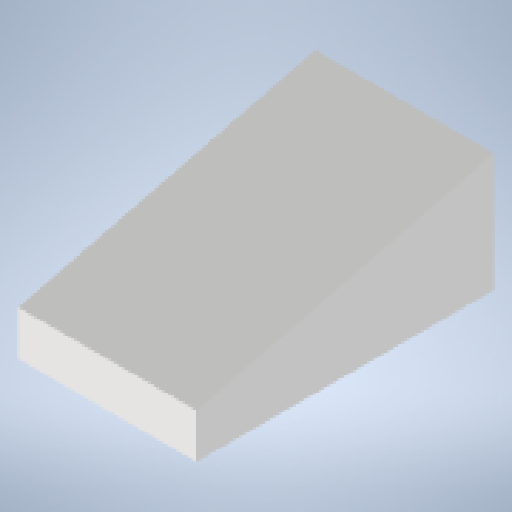
# Autodesk Inventor part: BeltClampNew
Saved by Autodesk Inventor 2023 (Build 270158000, 158)
## iProperties
Created: 2023-09-04
Part Number: BeltClampNew
Material: Generic
Document SubType Name: Modeling
Designer: Felix
Density: 1 g/cm^3
Appearance: Default
Author: Felix
Autodesk Inventor part; units mm, degrees
ref_plane "YZ Plane" through (0, 0, 0) normal (1, 0, 0) x (0, 1, 0)
ref_plane "XZ Plane" through (0, 0, 0) normal (0, 1, 0) x (-1, 0, 0)
ref_plane "XY Plane" through (0, 0, 0) normal (0, 0, 1) x (1, 0, 0)
sketch "Sketch1" plane through (0, 0, 0) normal (1, 0, 0) x (0, 1, 0)
  line L0 (0, 0) -> (0, -20)
  line L1 (0, -20) -> (8, -20)
  line L2 (8, -20) -> (3, 0)
  line L3 (3, 0) -> (0, 0)
  dimension "d0" = 8
  dimension "d1" = 20
  dimension "d11" = 3
  constraints: 8 end point, 2 perpendicular, 1 vertical
  measures "d0" distance of L0.end L1.end
  measures "d1" distance of L0.start L0.end
  measures "d11" distance of L2.end L0.start
extrude "Extrusion1" add sketch "Sketch1" along normal blind 12
sketch "Sketch2" plane through (0, 0, -20) normal (0, 0, -1) x (-1, 0, 0)
  line L0 (0, 0) -> (0, 8) construction
  line L1 (0, 8) -> (-12, 8) construction
  line L2 (-12, 0) -> (-12, 8) construction
  line L3 (0, 0) -> (-12, 0) construction
  line L4 (-12, 8) -> (0, 0) construction
  line L5 (0, 8) -> (-12, 0) construction
  point P0 (0, 0)
  point P1 (-6, 4)
  constraints: 4 end point, 1 midpoint
hole "Hole1" at (6, 4, -20) direction (0, 0, 1) diameter 4.3 depth 7
sketch "Sketch3" plane through (0, 0, 0) normal (-1, 0, 0) x (0, 0, 1)
  line L0 (-20, 0) -> (-20, 8) projected
  line L1 (-20, 8) -> (0, 3) projected
  line L2 (0, 3) -> (0, 0) projected
  line L3 (0, 0) -> (-20, 0) projected
  line L4 (-20, 15) -> (0, 15)
  line L5 (0, 15) -> (0, 5)
  line L6 (0, 5) -> (-20, 13.9197)
  line L7 (-20, 13.9197) -> (-20, 15)
  dimension "d12" = 15
  dimension "d13" = 2
  dimension "d14" = 10
  constraints: 8 end point, 2 vertical alignment, 1 horizontal, 1 parallel, 1 perpendicular
  measures "d12" distance between parallel lines of L3 L4
  measures "d13" distance of L1.end L5.end
  measures "d14" angle of L1 L6
extrude "Extrusion2" add sketch "Sketch3" against normal up to surface (12 mm away) contours L4 L5 L6 L7
sketch "Sketch4" plane through (0, 0, 0) normal (-1, 0, 0) x (0, 0, 1)
  line L0 (-20, 15) -> (-20, 13.9197) projected
  line L1 (0, 0) -> (-20, 0) projected
  line L2 (-20, 15) -> (0, 15)
  line L3 (0, 15) -> (0, 0)
  line L4 (0, 0) -> (-20, 0)
  line L5 (-20, 0) -> (-20, 15)
  constraints: 8 end point, 2 parallel, 1 horizontal, 1 perpendicular
extrude "Extrusion3" add sketch "Sketch4" along normal blind 2
sketch "Sketch5" plane through (12, 0, 0) normal (1, 0, 0) x (0, 0, -1)
  line L0 (0, 0) -> (0, 15) projected
  line L1 (0, 15) -> (20, 15) projected
  line L2 (0, 0) -> (20, 0)
  line L3 (20, 0) -> (20, 15)
  line L4 (20, 15) -> (0, 15)
  line L5 (0, 15) -> (0, 0)
  constraints: 8 end point, 2 parallel, 1 horizontal, 1 perpendicular
extrude "Extrusion4" add sketch "Sketch5" along normal blind 2
fillet "Fillet1" radius 2 2 edges at (-2, 15, -10) (14, 15, -10)
body "Solid1"
